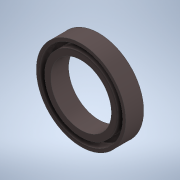
# Autodesk Inventor part: seal-ring-17x25x5
Saved by Autodesk Inventor 2022 (Build 260153000, 153)
## iProperties
Created: 2025-01-14
Part Number: seal-ring-17x25x5
Material: Generic
Document SubType Name: Modeling
Designer: Kostic
Density: 1 g/cm^3
Appearance: Default
Author: Kostic
Autodesk Inventor part; units mm, degrees
ref_plane "YZ Plane" through (0, 0, 0) normal (1, 0, 0) x (0, 1, 0)
ref_plane "XZ Plane" through (0, 0, 0) normal (0, 1, 0) x (-1, 0, 0)
ref_plane "XY Plane" through (0, 0, 0) normal (0, 0, 1) x (1, 0, 0)
sketch "Sketch1" plane through (0, 0, 0) normal (0, 0, 1) x (1, 0, 0)
  circle A0 centre (0, 0) radius 12.5
  circle A1 centre (0, 0) radius 8.5
  dimension "d0" = 25
  dimension "d1" = 17
  constraints: 2 centre point, 2 coincident
  measures "d0" diameter of A0
  measures "d1" diameter of A1
extrude "Extrusion1" add sketch "Sketch1" along normal blind 5
sketch "Sketch2" plane through (0, 0, 5) normal (0, 0, 1) x (1, 0, 0)
  circle A0 centre (0, 0) radius 12.5 projected
  circle A1 centre (0, 0) radius 8.5 projected
  circle A2 centre (0, 0) radius 11.6035
  circle A3 centre (0, 0) radius 10.2199
  constraints: 2 centre point
extrude "Extrusion2" cut sketch "Sketch2" against normal blind 3 contours A2
body "Solid1"
